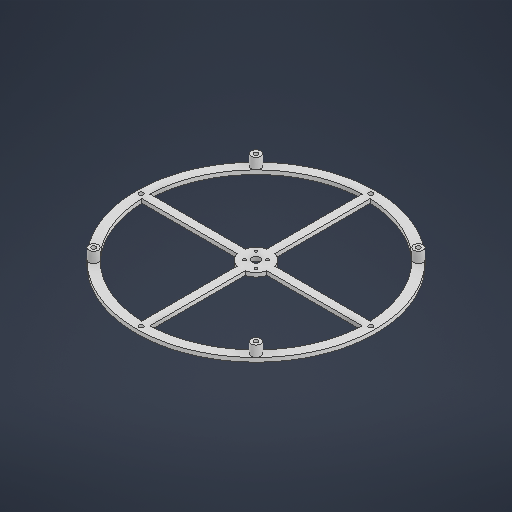
# Autodesk Inventor part: rama-silnik-gora-1
Saved by Autodesk Inventor 2026.2 (Build 302298010, 298A)
## iProperties
Created: 2026-04-17
Part Number: rama-silnik-gora-1
Material: Ogólny
Document SubType Name: Modeling
Designer: macie
Density: 1 g/cm^3
Appearance: Domyślna
Author: macie
Autodesk Inventor part; units mm, degrees
ref_plane "YZ Plane" through (0, 0, 0) normal (1, 0, 0) x (0, 1, 0)
ref_plane "XZ Plane" through (0, 0, 0) normal (0, 1, 0) x (-1, 0, 0)
ref_plane "XY Plane" through (0, 0, 0) normal (0, 0, 1) x (1, 0, 0)
sketch "Szkic1" plane through (0, 0, 0) normal (0, 1, 0) x (-1, 0, 0)
  circle A0 centre (0, 0) radius 11.5
  circle A1 centre (0, 0) radius 3
  line L0 (6, 8) -> (-6, 8)
  line L1 (-6, 8) -> (-6, -8)
  line L2 (-6, -8) -> (6, -8)
  line L3 (6, -8) -> (6, 8)
  line L4 (6, 8) -> (-6, -8) construction
  line L5 (-6, 8) -> (6, -8) construction
  line L6 (0, 8) -> (6, 0)
  line L7 (6, 0) -> (0, -8)
  line L8 (0, -8) -> (-6, 0)
  line L9 (-6, 0) -> (0, 8)
  dimension "d0" = 23
  dimension "d1" = 6
  dimension "d2" = 16
  dimension "d3" = 12
  constraints: 20 end point, 6 midpoint, 3 parallel, 2 centre point, 2 coincident, 1 horizontal, 1 perpendicular
  measures "d0" diameter of A0
  measures "d1" diameter of A1
  measures "d2" distance between parallel lines of L0 L2
  measures "d3" distance between parallel lines of L3 L1
extrude "Wyciągnięcie proste1" add sketch "Szkic1" along normal blind 3 contours A0 | L3 L6 L0 | L9 L1 L0 | L6 L7 L8 L9 | L3 L2 L7 | L8 L2 L1
sketch "Szkic2" plane through (0, 0, 0) normal (0, -1, 0) x (1, 0, 0)
  circle A0 centre (0, 0) radius 11.5 projected
  line L0 (-11.5, 0) -> (-11.5, -3)
  line L1 (-11.5, -3) -> (-82.2, -3)
  line L2 (-82.2, -3) -> (-82.2, 3)
  line L3 (-82.2, 3) -> (-11.5, 3)
  line L4 (-11.5, 3) -> (-11.5, -3)
  line L5 (-11.5, 3) -> (-11.1018, 3)
  line L6 (-11.5, -3) -> (-11.1018, -3)
  circle A1 centre (0, 0) radius 3 projected
  line L7 (3, -11.5) -> (3, -82.2)
  line L8 (-3, -82.2) -> (-3, -11.5)
  line L9 (3, -11.5) -> (3, -11.1018)
  line L10 (0, -11.5) -> (3, -11.5)
  line L11 (-3, -11.5) -> (-3, -11.1018)
  line L12 (-3, -11.5) -> (3, -11.5)
  line L13 (3, -82.2) -> (-3, -82.2)
  line L14 (11.5, 3) -> (82.2, 3)
  line L15 (82.2, -3) -> (11.5, -3)
  line L16 (11.5, 3) -> (11.1018, 3)
  line L17 (11.5, 0) -> (11.5, 3)
  line L18 (11.5, -3) -> (11.1018, -3)
  line L19 (11.5, -3) -> (11.5, 3)
  line L20 (82.2, 3) -> (82.2, -3)
  line L21 (-3, 11.5) -> (-3, 82.2)
  line L22 (3, 82.2) -> (3, 11.5)
  line L23 (-3, 11.5) -> (-3, 11.1018)
  line L24 (0, 11.5) -> (-3, 11.5)
  line L25 (3, 11.5) -> (3, 11.1018)
  line L26 (3, 11.5) -> (-3, 11.5)
  line L27 (-3, 82.2) -> (3, 82.2)
  circle A2 centre (0, 0) radius 82.2547
  circle A3 centre (0, 0) radius 89.2547
  point P0 (-11.5, 0)
  point P1 (0, -11.5)
  point P2 (11.5, 0)
  point P3 (0, 11.5)
  point P4 (11.5, 0)
  point P5 (11.5, 0)
  point P6 (11.5, 0)
  dimension "d15" = 70.7
  dimension "d17" = 6
  dimension "d18" = 3
  dimension "d21" = 360
  dimension "d23" = 7
  constraints: 56 end point, 3 parallel, 3 point on circle, 2 coincident, 2 horizontal, 1 centre point, 1 midpoint, 1 perpendicular, 1 tangent, 1 vertical, 64 other
  measures "d15" distance between parallel lines of L2 L4
  measures "d17" distance between parallel lines of L3 L1
  measures "d18" distance from line of L0.start L3
extrude "Wyciągnięcie proste2" add sketch "Szkic2" against normal blind 3 contours L19 L18 A0 | A0 L16 L17 | L17 L14 L20 L15 L19 | A0 L26 L25 | L9 L10 A0 | A2 L20 | A0 L23 L24 | L24 L21 L27 L22 L26 | L12 L11 A0 | L10 L7 L13 L8 L12 | L27 A2 | A2 L13 | A0 L4 L5 | L6 L0 A0 | L3 L4 L0 L1 L2 | L2 A2 | A3
sketch "Szkic3" plane through (0, 3, 0) normal (0, 1, 0) x (1, 0, 0)
  line L0 (82.2, 3) -> (11.1018, 3) projected
  circle A0 centre (0, 0) radius 89.2547 projected
  line L1 (0, 89.2547) -> (89.2547, 89.2547)
  line L2 (89.2547, 89.2547) -> (89.2547, 0)
  line L3 (89.2547, 0) -> (0, 0)
  line L4 (0, 0) -> (0, 89.2547)
  circle A1 centre (0, 0) radius 3 projected
  line L5 (0, 0) -> (89.2547, 89.2547)
  circle A2 centre (60.6377, 60.6377) radius 3.5
  arc A3 (82.2, 3) -> (3, 82.2) centre (0, 0) ccw projected
  circle A4 centre (0, 85.7547) radius 3.5
  circle A5 centre (-60.6377, 60.6377) radius 3.5
  circle A6 centre (-85.7547, 0) radius 3.5
  circle A7 centre (-60.6377, -60.6377) radius 3.5
  circle A8 centre (0, -85.7547) radius 3.5
  circle A9 centre (60.6377, -60.6377) radius 3.5
  circle A10 centre (85.7547, 0) radius 3.5
  dimension "d42" = 360
  constraints: 10 end point, 8 centre point, 2 parallel, 2 point on circle, 2 tangent, 1 horizontal, 1 perpendicular, 1 point on line, 17 other
hole "Otwór3" at (60.6377, 3, -60.6377) at (0, 3, -85.7547) at (-60.6377, 3, -60.6377) at (-85.7547, 3, 0) at (85.7547, 3, 0) at (-60.6377, 3, 60.6377) at (0, 3, 85.7547) at (60.6377, 3, 60.6377) direction (0, -1, 0) diameter 3.2 end through all
sketch "Szkic4" plane through (0, 3, 0) normal (0, 1, 0) x (1, 0, 0)
  circle A0 centre (60.6377, 60.6377) radius 1.6 projected
  circle A1 centre (60.6377, 60.6377) radius 3.5
  arc A2 (82.2, 3) -> (3, 82.2) centre (0, 0) ccw projected
  circle A3 centre (60.6377, 60.6377) radius 1.6
  circle A4 centre (-60.6377, 60.6377) radius 3.5
  circle A5 centre (-60.6377, 60.6377) radius 1.6
  circle A6 centre (-60.6377, -60.6377) radius 3.5
  circle A7 centre (-60.6377, -60.6377) radius 1.6
  circle A8 centre (60.6377, -60.6377) radius 3.5
  circle A9 centre (60.6377, -60.6377) radius 1.6
  dimension "d53" = 360
  constraints: 8 centre point, 2 coincident, 1 concentric, 1 tangent, 17 other
extrude "Wyciągnięcie proste3" add sketch "Szkic4" along normal blind 8
sketch "Szkic5" plane through (0, 3, 0) normal (0, 1, 0) x (1, 0, 0)
  line L0 (9.8995, -1.4142) -> (1.4142, -9.8995)
  line L1 (1.4142, -9.8995) -> (-9.8995, 1.4142)
  line L2 (-9.8995, 1.4142) -> (-1.4142, 9.8995)
  line L3 (-1.4142, 9.8995) -> (9.8995, -1.4142)
  arc A0 (3, -11.1018) -> (11.1018, -3) centre (0, 0) ccw projected
  arc A1 (-11.1018, -3) -> (-3, -11.1018) centre (0, 0) ccw projected
  line L4 (3, -11.1018) -> (-3, -11.1018)
  line L5 (5.6569, -5.6569) -> (4.2426, 4.2426)
  line L6 (4.2426, 4.2426) -> (-5.6569, 5.6569)
  line L7 (-5.6569, 5.6569) -> (-4.2426, -4.2426)
  line L8 (-4.2426, -4.2426) -> (5.6569, -5.6569)
  dimension "d57" = 45
  dimension "d58" = 12
  dimension "d59" = 16
  dimension "d60" = 6
  dimension "d61" = 8
  constraints: 18 end point, 4 midpoint, 3 parallel, 1 horizontal, 1 perpendicular
  measures "d57" angle of L4 L3
  measures "d58" distance between parallel lines of L1 L3
  measures "d59" distance between parallel lines of L2 L0
  measures "d60" distance from line of L3 point (0, 0)
  measures "d61" distance from line of point (0, 0) L0
hole "Otwór4" at (5.6569, 3, 5.6569) at (4.2426, 3, -4.2426) at (-5.6569, 3, -5.6569) at (-4.2426, 3, 4.2426) direction (0, -1, 0) diameter 2.1 end through all
